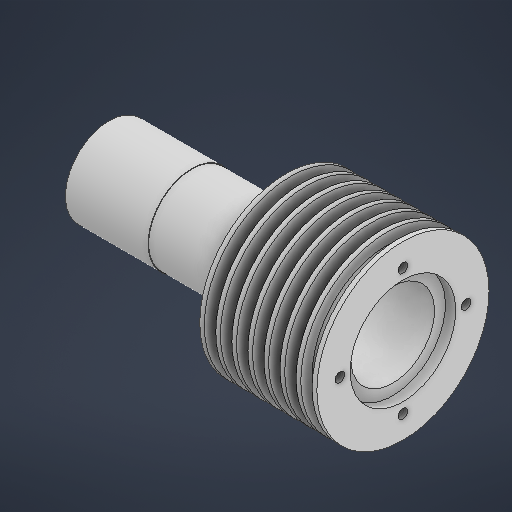
# Autodesk Inventor part: HeatExchangeCylinder
Saved by Autodesk Inventor 2025.4 (Build 294407000, 407)
## iProperties
Created: 2026-05-29
Part Number: HeatExchangeCylinder
Material: Generic
Document SubType Name: Modeling
Designer: VuQuan
Density: 1 g/cm^3
Appearance: Default
Author: VuQuan
Autodesk Inventor part; units mm, degrees
ref_plane "YZ Plane" through (0, 0, 0) normal (1, 0, 0) x (0, 1, 0)
ref_plane "XZ Plane" through (0, 0, 0) normal (0, 1, 0) x (-1, 0, 0)
ref_plane "XY Plane" through (0, 0, 0) normal (0, 0, 1) x (1, 0, 0)
sketch "Sketch1" plane through (0, 0, 0) normal (0, 0, 1) x (1, 0, 0)
  line L0 (0, 0) -> (164, 0) construction
  line L1 (0, 19) -> (36, 19)
  line L2 (0, 19) -> (0, 18.25)
  line L3 (0, 18.25) -> (123.5, 18.25)
  line L4 (123.5, 18.25) -> (123.5, 23)
  line L5 (123.5, 23) -> (128, 23)
  line L6 (128, 23) -> (128, 37.5)
  line L7 (128, 37.5) -> (126, 37.5)
  line L8 (126, 37.5) -> (126, 32.5255)
  line L9 (36, 19) -> (36, 18.75)
  line L10 (36, 18.75) -> (72, 18.75)
  line L11 (72, 18.75) -> (72, 19)
  line L12 (72, 19) -> (77, 19)
  line L13 (77, 19) -> (77, 37.5)
  line L14 (77, 37.5) -> (79, 37.5)
  line L15 (79, 37.5) -> (79, 19)
  line L16 (79, 19) -> (84, 19)
  line L17 (84, 19) -> (84, 37.5)
  line L18 (84, 37.5) -> (86, 37.5)
  line L19 (86, 37.5) -> (86, 19)
  line L20 (86, 19) -> (91, 19)
  line L21 (91, 19) -> (91, 37.5)
  line L22 (91, 37.5) -> (93, 37.5)
  line L23 (93, 37.5) -> (93, 19)
  line L24 (93, 19) -> (98, 19)
  line L25 (98, 19) -> (98, 37.5)
  line L26 (98, 37.5) -> (100, 37.5)
  line L27 (100, 37.5) -> (100, 19)
  line L28 (100, 19) -> (105, 19)
  line L29 (105, 19) -> (105, 37.5)
  line L30 (105, 37.5) -> (107, 37.5)
  line L31 (107, 37.5) -> (107, 19)
  line L32 (107, 19) -> (112, 19)
  line L33 (112, 19) -> (112, 37.5)
  line L34 (112, 37.5) -> (114, 37.5)
  line L35 (114, 37.5) -> (114, 19)
  line L36 (114, 19) -> (119, 19)
  line L37 (126, 32.5255) -> (121, 32.5255)
  line L38 (121, 32.5255) -> (121, 37.5)
  line L39 (121, 37.5) -> (119, 37.5)
  line L40 (119, 37.5) -> (119, 19)
  point P0 (123.5, 32.5255)
  dimension "d0" = 38
  dimension "d1" = 36.5
  dimension "d2" = 46
  dimension "d3" = 37.5
  dimension "d4" = 36
  dimension "d5" = 36
  dimension "d6" = 2
  dimension "d7" = 75
  dimension "d10" = 7
  dimension "d15" = 9
  dimension "d16" = 128
  constraints: 82 end point, 13 perpendicular, 6 collinear, 5 vertical, 4 horizontal, 3 point on line, 1 midpoint, 45 other
  measures "d0" diameter of L1 L0
  measures "d1" diameter of L3 L0
  measures "d2" diameter of L5 L0
  measures "d3" diameter of L10 L0
  measures "d4" distance of L1.start L1.end
  measures "d5" distance of L9.end L10.end
  measures "d6" distance between parallel lines of L15 L13
  measures "d7" diameter of L14 L0
  measures "d10" distance of L12.end L17.start
  measures "d15" distance between parallel lines of L6 L40
  measures "d16" distance from line of L0.start L6
revolve "Revolution1" add sketch "Sketch1" angle 360 about axis through (0, 0, 0) along (1, 0, 0)
sketch "Sketch2" plane through (128, 0, 0) normal (1, 0, 0) x (0, 0, -1)
  circle A0 centre (0, 0) radius 37.5 projected
  circle A1 centre (0, 0) radius 23 projected
  circle A2 centre (0, 0) radius 27.5 construction
  point P0 (0, 27.5)
  point P1 (-27.5, 0)
  point P2 (0, -27.5)
  point P3 (27.5, 0)
  dimension "d18" = 55
  dimension "d21" = 360
  constraints: 2 vertical alignment, 1 coincident, 7 other
hole "Hole1" at (128, 27.5, 0) at (128, 0, -27.5) at (128, -27.5, 0) at (128, 0, 27.5) direction (-1, 0, 0) diameter 4.134 depth 9 thread size "M5x0.8" class "6H" standard "ISO Metric profile"
body "Solid1"
